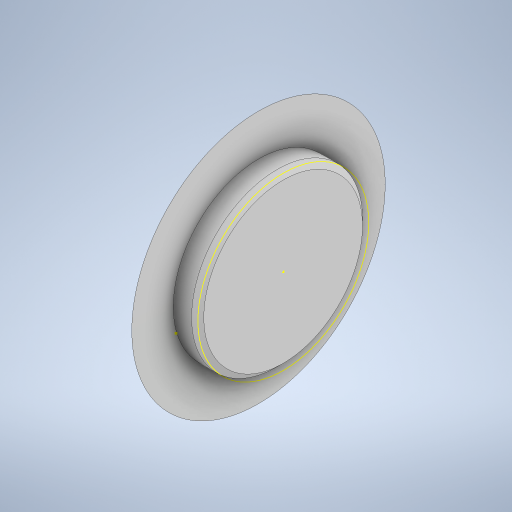
# Autodesk Inventor part: Poklopac VV
Saved by Autodesk Inventor 2024.2 (Build 282272000, 272)
## iProperties
Created: 2024-06-04
Part Number: Poklopac VV
Material: Generic
Document SubType Name: Modeling
Designer: ljubopudar
Density: 1 g/cm^3
Appearance: Default
Author: ljubopudar
Autodesk Inventor part; units mm, degrees
ref_plane "YZ Plane" through (0, 0, 0) normal (1, 0, 0) x (0, 1, 0)
ref_plane "XZ Plane" through (0, 0, 0) normal (0, 1, 0) x (-1, 0, 0)
ref_plane "XY Plane" through (0, 0, 0) normal (0, 0, 1) x (1, 0, 0)
sketch "Sketch1" plane through (0, 0, 0) normal (0, 1, 0) x (-1, 0, 0)
  line L0 (196.8659, -17.545) -> (196.8659, -26.6873)
  line L1 (196.8659, -17.545) -> (228.8659, -17.545)
  line L2 (227.7626, -32.3076) -> (197.7136, -27.6756)
  line L3 (228.8659, -17.545) -> (246.8659, -17.545)
  line L4 (246.8659, -17.545) -> (237.6813, -17.545)
  line L5 (246.8659, -17.545) -> (245.8659, -17.545)
  arc A0 (196.8659, -26.6873) -> (197.7136, -27.6756) centre (197.8659, -26.6873) ccw
  line L6 (196.8659, -17.545) -> (246.8659, -17.545)
  arc A1 (229.126, -33.1809) -> (227.7626, -32.3076) centre (227.4579, -34.2842) ccw
  ellipse E0 centre (237.6813, -17.545) end of major axis (237.5408, 7.368) minor radius 11.0798 (229.126, -33.1809) -> (248.7612, -17.545) ccw
  line L7 (244.9773, -17.545) -> (255.0074, -17.545)
  line L8 (196.8659, -17.545) -> (230.8659, -17.545)
  line L9 (230.8659, -17.545) -> (230.8659, -31.545)
  line L10 (230.8659, -31.545) -> (243.8659, -31.545)
  line L11 (243.8659, -31.545) -> (243.9734, -50.6163)
  line L12 (243.9734, -50.6163) -> (189.9341, -50.921)
  line L13 (189.9341, -50.921) -> (189.7459, -17.545)
  line L14 (189.7459, -17.545) -> (196.8659, -17.545)
  line L15 (243.8659, -31.545) -> (239.8659, -31.545)
  line L16 (239.8659, -31.545) -> (239.8659, -17.545)
  point P0 (0, 0)
  point P1 (196.8659, -27.545)
  point P2 (236.8686, -42.545)
  point P3 (196.8659, -22.1161)
  point P4 (237.8659, -17.545)
  point P5 (300.0729, -77.6732)
  point P6 (243.904, -38.2995)
  point P7 (248.7612, -17.545)
  dimension "d26" = 11.0798
  dimension "d20" = 10
  dimension "d21" = 1
  dimension "d22" = 25
  dimension "d23" = 2
  dimension "d24" = 16.7393
  dimension "d25" = 30.592
  dimension "d27" = 41
  dimension "d28" = 11.08
  dimension "d33" = 34
  dimension "d34" = 14
  dimension "d35" = 13
  dimension "d36" = 4
  constraints: 34 end point, 12 point on line, 4 perpendicular, 4 point on circle, 3 tangent, 2 centre point, 2 midpoint, 1 coincident, 1 collinear, 1 horizontal, 1 parallel, 1 vertical, 5 other
  measures "d20" distance of L0.start point (196.866, -27.545)
  measures "d21" radius of A0
  measures "d22" vertical distance of L4.end point (236.869, -42.545)
  measures "d23" radius of A1
  measures "d24" distance from line of L1 A1.centre
  measures "d25" distance from line of L0 A1.centre
  measures "d27" distance of point (237.866, -17.545) L0.start
  measures "d28" distance of point (248.761, -17.545) L4.end
  measures "d33" distance of L0.start L8.end
  measures "d34" distance of L8.end L9.end
  measures "d35" distance of L9.end L10.end
  measures "d36" distance of L10.end L15.end
revolve "Revolution3" add sketch "Sketch1" angle 360 about axis through (-228.8659, 0, -17.545) along (-1, 0, 0) contours L3 L7 E0 L11 L10 L16
chamfer "Chamfer2" distance 1 angle 45 1 edges at (-239.8659, 0, -3.545)
sketch "Sketch2" plane through (-239.8659, 0, -17.545) normal (1, 0, 0) x (0, 0, -1)
  circle A0 centre (0, 0) radius 14 projected
  point P0 (-17.545, 0)
body "Solid2"
